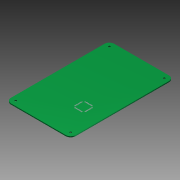
# Autodesk Inventor part: Base station. Board
Saved by Autodesk Inventor 2011 (Build 150239000, 239)
## iProperties
Created: 2011-04-11
Part Number: Base station. Board
Document SubType Name: Modeling
Designer: Rob
Density: 1 g/cm^3
Author: Rob
Autodesk Inventor part; units mm, degrees
ref_plane "YZ Plane" through (0, 0, 0) normal (1, 0, 0) x (0, 1, 0)
ref_plane "XZ Plane" through (0, 0, 0) normal (0, 1, 0) x (-1, 0, 0)
ref_plane "XY Plane" through (0, 0, 0) normal (0, 0, 1) x (1, 0, 0)
sketch "Sketch1" plane through (0, 0, 0) normal (0, 0, 1) x (1, 0, 0)
  line L0 (-50, 80) -> (50, 80)
  line L1 (50, 80) -> (50, -80)
  line L2 (50, -80) -> (-50, -80)
  line L3 (-50, -80) -> (-50, 80)
  line L4 (0, 0) -> (5.0771, 0)
  line L5 (0, 0) -> (0, -4.8823)
  dimension "d0" = 100
  dimension "d1" = 160
  constraints: 12 end point, 3 perpendicular, 2 parallel, 1 horizontal, 2 other
  measures "d0" distance of L1.end L2.end
  measures "d1" distance of L0.end L1.end
extrude "Extrusion1" add sketch "Sketch1" along normal blind 1.6
fillet "Fillet1" radius 7.5 4 edges at (-50, -80, 0.8) (50, -80, 0.8) (-50, 80, 0.8) (50, 80, 0.8)
sketch "Sketch2" plane through (0, 0, 1.6) normal (0, 0, 1) x (1, 0, 0)
  arc A0 (50, 72.5) -> (42.5, 80) centre (42.5, 72.5) ccw projected
  arc A1 (-42.5, 80) -> (-50, 72.5) centre (-42.5, 72.5) ccw projected
  arc A2 (-50, -72.5) -> (-42.5, -80) centre (-42.5, -72.5) ccw projected
  arc A3 (42.5, -80) -> (50, -72.5) centre (42.5, -72.5) ccw projected
  circle A4 centre (-42.5, 72.5) radius 1.5
  circle A5 centre (-42.5, -72.5) radius 1.5
  circle A6 centre (42.5, -72.5) radius 1.5
  circle A7 centre (42.5, 72.5) radius 1.5
  point P0 (0, 0)
  dimension "d5" = 3
  dimension "d6" = 3
  dimension "d7" = 3
  dimension "d8" = 3
  constraints: 4 centre point, 4 coincident
  measures "d5" diameter of A4
  measures "d6" diameter of A5
  measures "d7" diameter of A6
  measures "d8" diameter of A7
extrude "Extrusion2" cut sketch "Sketch2" against normal through all
sketch "Sketch4" plane through (0, 0, 1.6) normal (0, 0, 1) x (1, 0, 0)
  line L0 (42.5, -80) -> (-42.5, -80) projected
  line L1 (50, 72.5) -> (50, -72.5) projected
  line L2 (9.5, -37) -> (27, -37)
  line L3 (27, -37) -> (27, -19.5)
  line L4 (27, -19.5) -> (9.5, -19.5)
  line L5 (9.5, -19.5) -> (9.5, -37)
  line L6 (12.25, -35.25) -> (24.25, -35.25)
  line L7 (25.25, -34.25) -> (25.25, -22.25)
  line L8 (24.25, -21.25) -> (12.25, -21.25)
  line L9 (11.25, -22.25) -> (11.25, -34.25)
  line L10 (18.25, -31.1458) -> (18.25, -23.2964)
  line L11 (18.25, -28.25) -> (14.0823, -28.25)
  arc A0 (11.25, -34.25) -> (12.25, -35.25) centre (12.25, -34.25) ccw
  arc A1 (12.25, -21.25) -> (11.25, -22.25) centre (12.25, -22.25) ccw
  arc A2 (25.25, -22.25) -> (24.25, -21.25) centre (24.25, -22.25) ccw
  arc A3 (24.25, -35.25) -> (25.25, -34.25) centre (24.25, -34.25) ccw
  line L12 (12.25, -21.25) -> (12.75, -21.25)
  line L13 (12.75, -21.25) -> (12.75, -19.5)
  line L14 (12.75, -19.5) -> (12.25, -19.5)
  line L15 (12.25, -19.5) -> (12.25, -21.25)
  line L16 (24.25, -21.25) -> (23.75, -21.25)
  line L17 (23.75, -19.5) -> (24.25, -19.5)
  line L18 (13.0167, -21.25) -> (13.5167, -21.25)
  line L19 (13.5167, -21.25) -> (13.5167, -19.5)
  line L20 (13.5167, -19.5) -> (13.0167, -19.5)
  line L21 (13.0167, -19.5) -> (13.0167, -21.25)
  line L22 (18.1167, -21.25) -> (17.6167, -21.25)
  line L23 (17.6167, -21.25) -> (17.6167, -19.5)
  line L24 (17.6167, -19.5) -> (18.1167, -19.5)
  line L25 (18.1167, -19.5) -> (18.1167, -21.25)
  line L26 (13.7833, -21.25) -> (14.2833, -21.25)
  line L27 (14.2833, -21.25) -> (14.2833, -19.5)
  line L28 (14.2833, -19.5) -> (13.7833, -19.5)
  line L29 (13.7833, -19.5) -> (13.7833, -21.25)
  line L30 (14.55, -21.25) -> (15.05, -21.25)
  line L31 (15.05, -21.25) -> (15.05, -19.5)
  line L32 (15.05, -19.5) -> (14.55, -19.5)
  line L33 (14.55, -19.5) -> (14.55, -21.25)
  line L34 (15.3167, -21.25) -> (15.8167, -21.25)
  line L35 (15.8167, -21.25) -> (15.8167, -19.5)
  line L36 (15.8167, -19.5) -> (15.3167, -19.5)
  line L37 (15.3167, -19.5) -> (15.3167, -21.25)
  line L38 (16.0833, -21.25) -> (16.5833, -21.25)
  line L39 (16.5833, -21.25) -> (16.5833, -19.5)
  line L40 (16.5833, -19.5) -> (16.0833, -19.5)
  line L41 (16.0833, -19.5) -> (16.0833, -21.25)
  line L42 (16.85, -21.25) -> (17.35, -21.25)
  line L43 (17.35, -21.25) -> (17.35, -19.5)
  line L44 (17.35, -19.5) -> (16.85, -19.5)
  line L45 (16.85, -19.5) -> (16.85, -21.25)
  line L46 (24.25, -21.25) -> (23.75, -21.25)
  line L47 (23.75, -21.25) -> (23.75, -19.5)
  line L48 (23.75, -19.5) -> (24.25, -19.5)
  line L49 (24.25, -19.5) -> (24.25, -21.25)
  line L50 (23.4833, -21.25) -> (22.9833, -21.25)
  line L51 (22.9833, -21.25) -> (22.9833, -19.5)
  line L52 (22.9833, -19.5) -> (23.4833, -19.5)
  line L53 (23.4833, -19.5) -> (23.4833, -21.25)
  line L54 (18.3833, -21.25) -> (18.8833, -21.25)
  line L55 (18.8833, -21.25) -> (18.8833, -19.5)
  line L56 (18.8833, -19.5) -> (18.3833, -19.5)
  line L57 (18.3833, -19.5) -> (18.3833, -21.25)
  line L58 (22.7167, -21.25) -> (22.2167, -21.25)
  line L59 (22.2167, -21.25) -> (22.2167, -19.5)
  line L60 (22.2167, -19.5) -> (22.7167, -19.5)
  line L61 (22.7167, -19.5) -> (22.7167, -21.25)
  line L62 (21.95, -21.25) -> (21.45, -21.25)
  line L63 (21.45, -21.25) -> (21.45, -19.5)
  line L64 (21.45, -19.5) -> (21.95, -19.5)
  line L65 (21.95, -19.5) -> (21.95, -21.25)
  line L66 (21.1833, -21.25) -> (20.6833, -21.25)
  line L67 (20.6833, -21.25) -> (20.6833, -19.5)
  line L68 (20.6833, -19.5) -> (21.1833, -19.5)
  line L69 (21.1833, -19.5) -> (21.1833, -21.25)
  line L70 (20.4167, -21.25) -> (19.9167, -21.25)
  line L71 (19.9167, -21.25) -> (19.9167, -19.5)
  line L72 (19.9167, -19.5) -> (20.4167, -19.5)
  line L73 (20.4167, -19.5) -> (20.4167, -21.25)
  line L74 (19.65, -21.25) -> (19.15, -21.25)
  line L75 (19.15, -21.25) -> (19.15, -19.5)
  line L76 (19.15, -19.5) -> (19.65, -19.5)
  line L77 (19.65, -19.5) -> (19.65, -21.25)
  line L78 (24.25, -35.25) -> (12.25, -35.25)
  line L79 (12.25, -35.25) -> (12.75, -35.25)
  line L80 (12.75, -35.25) -> (12.75, -37)
  line L81 (12.75, -37) -> (12.25, -37)
  line L82 (12.25, -37) -> (12.25, -35.25)
  line L83 (24.25, -35.25) -> (23.75, -35.25)
  line L84 (23.75, -37) -> (24.25, -37)
  line L85 (13.0167, -35.25) -> (13.5167, -35.25)
  line L86 (13.5167, -35.25) -> (13.5167, -37)
  line L87 (13.5167, -37) -> (13.0167, -37)
  line L88 (13.0167, -37) -> (13.0167, -35.25)
  line L89 (18.1167, -35.25) -> (17.6167, -35.25)
  line L90 (17.6167, -35.25) -> (17.6167, -37)
  line L91 (17.6167, -37) -> (18.1167, -37)
  line L92 (18.1167, -37) -> (18.1167, -35.25)
  line L93 (13.7833, -35.25) -> (14.2833, -35.25)
  line L94 (14.2833, -35.25) -> (14.2833, -37)
  line L95 (14.2833, -37) -> (13.7833, -37)
  line L96 (13.7833, -37) -> (13.7833, -35.25)
  line L97 (14.55, -35.25) -> (15.05, -35.25)
  line L98 (15.05, -35.25) -> (15.05, -37)
  line L99 (15.05, -37) -> (14.55, -37)
  line L100 (14.55, -37) -> (14.55, -35.25)
  line L101 (15.3167, -35.25) -> (15.8167, -35.25)
  line L102 (15.8167, -35.25) -> (15.8167, -37)
  line L103 (15.8167, -37) -> (15.3167, -37)
  line L104 (15.3167, -37) -> (15.3167, -35.25)
  line L105 (16.0833, -35.25) -> (16.5833, -35.25)
  line L106 (16.5833, -35.25) -> (16.5833, -37)
  line L107 (16.5833, -37) -> (16.0833, -37)
  line L108 (16.0833, -37) -> (16.0833, -35.25)
  line L109 (16.85, -35.25) -> (17.35, -35.25)
  line L110 (17.35, -35.25) -> (17.35, -37)
  line L111 (17.35, -37) -> (16.85, -37)
  line L112 (16.85, -37) -> (16.85, -35.25)
  line L113 (21.95, -37) -> (21.95, -35.25)
  line L114 (21.45, -37) -> (21.95, -37)
  line L115 (21.95, -35.25) -> (21.45, -35.25)
  line L116 (21.1833, -35.25) -> (20.6833, -35.25)
  line L117 (21.1833, -37) -> (21.1833, -35.25)
  line L118 (20.6833, -35.25) -> (20.6833, -37)
  line L119 (20.6833, -37) -> (21.1833, -37)
  line L120 (21.45, -35.25) -> (21.45, -37)
  line L121 (18.3833, -35.25) -> (18.8833, -35.25)
  line L122 (19.65, -35.25) -> (19.15, -35.25)
  line L123 (20.4167, -35.25) -> (19.9167, -35.25)
  line L124 (18.8833, -35.25) -> (18.8833, -37)
  line L125 (18.8833, -37) -> (18.3833, -37)
  line L126 (18.3833, -37) -> (18.3833, -35.25)
  line L127 (19.15, -35.25) -> (19.15, -37)
  line L128 (19.65, -37) -> (19.65, -35.25)
  line L129 (19.15, -37) -> (19.65, -37)
  line L130 (19.9167, -35.25) -> (19.9167, -37)
  line L131 (20.4167, -37) -> (20.4167, -35.25)
  line L132 (19.9167, -37) -> (20.4167, -37)
  line L133 (24.25, -35.25) -> (23.75, -35.25)
  line L134 (23.75, -35.25) -> (23.75, -37)
  line L135 (23.75, -37) -> (24.25, -37)
  line L136 (22.2167, -35.25) -> (22.2167, -37)
  line L137 (22.7167, -35.25) -> (22.2167, -35.25)
  line L138 (22.2167, -37) -> (22.7167, -37)
  line L139 (22.7167, -37) -> (22.7167, -35.25)
  line L140 (22.9833, -35.25) -> (22.9833, -37)
  line L141 (22.9833, -37) -> (23.4833, -37)
  line L142 (23.4833, -37) -> (23.4833, -35.25)
  line L143 (24.25, -37) -> (24.25, -35.25)
  line L144 (23.4833, -35.25) -> (22.9833, -35.25)
  line L145 (11.25, -34.25) -> (9.5, -34.25)
  line L146 (9.5, -34.25) -> (9.5, -33.75)
  line L147 (9.5, -33.75) -> (11.25, -33.75)
  line L148 (11.25, -33.75) -> (11.25, -34.25)
  line L149 (9.5, -33.4833) -> (11.25, -33.4833)
  line L150 (11.25, -33.4833) -> (11.25, -32.9833)
  line L151 (11.25, -32.9833) -> (9.5, -32.9833)
  line L152 (9.5, -32.9833) -> (9.5, -33.4833)
  line L153 (9.5, -32.7167) -> (11.25, -32.7167)
  line L154 (11.25, -32.7167) -> (11.25, -32.2167)
  line L155 (11.25, -32.2167) -> (9.5, -32.2167)
  line L156 (9.5, -32.2167) -> (9.5, -32.7167)
  line L157 (9.5, -31.95) -> (11.25, -31.95)
  line L158 (11.25, -31.95) -> (11.25, -31.45)
  line L159 (11.25, -31.45) -> (9.5, -31.45)
  line L160 (9.5, -31.45) -> (9.5, -31.95)
  line L161 (9.5, -31.1833) -> (11.25, -31.1833)
  line L162 (11.25, -31.1833) -> (11.25, -30.6833)
  line L163 (11.25, -30.6833) -> (9.5, -30.6833)
  line L164 (9.5, -30.6833) -> (9.5, -31.1833)
  line L165 (9.5, -30.4167) -> (11.25, -30.4167)
  line L166 (11.25, -30.4167) -> (11.25, -29.9167)
  line L167 (11.25, -29.9167) -> (9.5, -29.9167)
  line L168 (9.5, -29.9167) -> (9.5, -30.4167)
  line L169 (9.5, -29.65) -> (11.25, -29.65)
  line L170 (11.25, -29.65) -> (11.25, -29.15)
  line L171 (11.25, -29.15) -> (9.5, -29.15)
  line L172 (9.5, -29.15) -> (9.5, -29.65)
  line L173 (9.5, -28.8833) -> (11.25, -28.8833)
  line L174 (11.25, -28.8833) -> (11.25, -28.3833)
  line L175 (11.25, -28.3833) -> (9.5, -28.3833)
  line L176 (9.5, -28.3833) -> (9.5, -28.8833)
  line L177 (11.25, -22.25) -> (9.5, -22.25)
  line L178 (9.5, -22.25) -> (9.5, -22.75)
  line L179 (9.5, -22.75) -> (11.25, -22.75)
  line L180 (11.25, -22.75) -> (11.25, -22.25)
  line L181 (9.5, -23.0167) -> (11.25, -23.0167)
  line L182 (11.25, -23.0167) -> (11.25, -23.5167)
  line L183 (11.25, -23.5167) -> (9.5, -23.5167)
  line L184 (9.5, -23.5167) -> (9.5, -23.0167)
  line L185 (9.5, -23.7833) -> (11.25, -23.7833)
  line L186 (11.25, -23.7833) -> (11.25, -24.2833)
  line L187 (11.25, -24.2833) -> (9.5, -24.2833)
  line L188 (9.5, -24.2833) -> (9.5, -23.7833)
  line L189 (9.5, -24.55) -> (11.25, -24.55)
  line L190 (11.25, -24.55) -> (11.25, -25.05)
  line L191 (11.25, -25.05) -> (9.5, -25.05)
  line L192 (9.5, -25.05) -> (9.5, -24.55)
  line L193 (9.5, -25.3167) -> (11.25, -25.3167)
  line L194 (11.25, -25.3167) -> (11.25, -25.8167)
  line L195 (11.25, -25.8167) -> (9.5, -25.8167)
  line L196 (9.5, -25.8167) -> (9.5, -25.3167)
  line L197 (9.5, -26.0833) -> (11.25, -26.0833)
  line L198 (11.25, -26.0833) -> (11.25, -26.5833)
  line L199 (11.25, -26.5833) -> (9.5, -26.5833)
  line L200 (9.5, -26.5833) -> (9.5, -26.0833)
  line L201 (9.5, -26.85) -> (11.25, -26.85)
  line L202 (11.25, -26.85) -> (11.25, -27.35)
  line L203 (11.25, -27.35) -> (9.5, -27.35)
  line L204 (9.5, -27.35) -> (9.5, -26.85)
  line L205 (9.5, -27.6167) -> (11.25, -27.6167)
  line L206 (11.25, -27.6167) -> (11.25, -28.1167)
  line L207 (11.25, -28.1167) -> (9.5, -28.1167)
  line L208 (9.5, -28.1167) -> (9.5, -27.6167)
  line L209 (25.25, -22.25) -> (25.25, -34.25)
  line L210 (25.25, -34.25) -> (27, -34.25)
  line L211 (27, -34.25) -> (27, -33.75)
  line L212 (27, -33.75) -> (25.25, -33.75)
  line L213 (25.25, -33.75) -> (25.25, -34.25)
  line L214 (27, -33.4833) -> (25.25, -33.4833)
  line L215 (25.25, -33.4833) -> (25.25, -32.9833)
  line L216 (25.25, -32.9833) -> (27, -32.9833)
  line L217 (27, -32.9833) -> (27, -33.4833)
  line L218 (27, -32.7167) -> (25.25, -32.7167)
  line L219 (25.25, -32.7167) -> (25.25, -32.2167)
  line L220 (25.25, -32.2167) -> (27, -32.2167)
  line L221 (27, -32.2167) -> (27, -32.7167)
  line L222 (27, -31.95) -> (25.25, -31.95)
  line L223 (25.25, -31.95) -> (25.25, -31.45)
  line L224 (25.25, -31.45) -> (27, -31.45)
  line L225 (27, -31.45) -> (27, -31.95)
  line L226 (27, -31.1833) -> (25.25, -31.1833)
  line L227 (25.25, -31.1833) -> (25.25, -30.6833)
  line L228 (25.25, -30.6833) -> (27, -30.6833)
  line L229 (27, -30.6833) -> (27, -31.1833)
  line L230 (27, -30.4167) -> (25.25, -30.4167)
  line L231 (25.25, -30.4167) -> (25.25, -29.9167)
  line L232 (25.25, -29.9167) -> (27, -29.9167)
  line L233 (27, -29.9167) -> (27, -30.4167)
  line L234 (27, -29.65) -> (25.25, -29.65)
  line L235 (25.25, -29.65) -> (25.25, -29.15)
  line L236 (25.25, -29.15) -> (27, -29.15)
  line L237 (27, -29.15) -> (27, -29.65)
  line L238 (27, -28.8833) -> (25.25, -28.8833)
  line L239 (25.25, -28.8833) -> (25.25, -28.3833)
  line L240 (25.25, -28.3833) -> (27, -28.3833)
  line L241 (27, -28.3833) -> (27, -28.8833)
  line L242 (25.25, -22.75) -> (25.25, -22.25)
  line L243 (25.25, -23.0167) -> (25.25, -23.5167)
  line L244 (27, -22.25) -> (27, -22.75)
  line L245 (27, -22.75) -> (25.25, -22.75)
  line L246 (27, -23.0167) -> (25.25, -23.0167)
  line L247 (25.25, -23.7833) -> (25.25, -24.2833)
  line L248 (27, -23.5167) -> (27, -23.0167)
  line L249 (25.25, -23.5167) -> (27, -23.5167)
  line L250 (27, -23.7833) -> (25.25, -23.7833)
  line L251 (25.25, -24.2833) -> (27, -24.2833)
  line L252 (27, -24.2833) -> (27, -23.7833)
  line L253 (27, -24.55) -> (25.25, -24.55)
  line L254 (25.25, -22.25) -> (27, -22.25)
  line L255 (25.25, -24.55) -> (25.25, -25.05)
  line L256 (25.25, -25.05) -> (27, -25.05)
  line L257 (27, -25.3167) -> (25.25, -25.3167)
  line L258 (25.25, -25.3167) -> (25.25, -25.8167)
  line L259 (25.25, -25.8167) -> (27, -25.8167)
  line L260 (27, -25.8167) -> (27, -25.3167)
  line L261 (27, -26.0833) -> (25.25, -26.0833)
  line L262 (25.25, -26.0833) -> (25.25, -26.5833)
  line L263 (27, -26.5833) -> (27, -26.0833)
  line L264 (27, -25.05) -> (27, -24.55)
  line L265 (25.25, -26.5833) -> (27, -26.5833)
  line L266 (27, -26.85) -> (25.25, -26.85)
  line L267 (25.25, -26.85) -> (25.25, -27.35)
  line L268 (27, -27.35) -> (27, -26.85)
  line L269 (25.25, -27.35) -> (27, -27.35)
  line L270 (27, -27.6167) -> (25.25, -27.6167)
  line L271 (25.25, -28.1167) -> (27, -28.1167)
  line L272 (27, -28.1167) -> (27, -27.6167)
  line L273 (25.25, -27.6167) -> (25.25, -28.1167)
  line L274 (18.1167, -19.5) -> (18.1167, -21.25)
  point P0 (0, 0)
  point P1 (25.25, -21.25)
  point P2 (25.25, -35.25)
  point P3 (11.25, -21.25)
  dimension "d11" = 17.5
  dimension "d12" = 17.5
  dimension "d13" = 23
  dimension "d14" = 43
  dimension "d15" = 14
  dimension "d16" = 14
  dimension "d17" = 1
  dimension "d18" = 0.5
  dimension "d19" = 0.5
  dimension "d20" = 0.5
  dimension "d21" = 0.5
  dimension "d22" = 0.5
  dimension "d23" = 0.5
  dimension "d24" = 0.5
  dimension "d25" = 0.5
  dimension "d26" = 0.5
  dimension "d27" = 0.2667
  dimension "d28" = 0.2667
  dimension "d29" = 0.2667
  dimension "d30" = 0.2667
  dimension "d31" = 0.2667
  dimension "d32" = 0.2667
  dimension "d33" = 0.2667
  dimension "d34" = 0.5
  dimension "d35" = 0.5
  dimension "d36" = 0.5
  dimension "d37" = 0.5
  dimension "d38" = 0.5
  dimension "d39" = 0.5
  dimension "d40" = 0.5
  dimension "d41" = 0.5
  dimension "d42" = 0.2667
  dimension "d43" = 0.2667
  dimension "d44" = 0.2667
  dimension "d45" = 0.2667
  dimension "d46" = 0.2667
  dimension "d47" = 0.2667
  dimension "d48" = 0.2667
  constraints: 534 end point, 183 symmetric about line, 37 parallel, 21 horizontal, 20 perpendicular, 8 point on circle, 5 point on line, 4 centre point, 4 tangent, 3 equal radius, 3 vertical, 70 other
  measures "d11" distance of point (9.5, -19.5) L3.end
  measures "d12" distance of L3.end L2.end
  measures "d13" distance between parallel lines of L3 L1
  measures "d14" distance between parallel lines of L0 L2
  measures "d15" distance of point (11.25, -21.25) point (25.25, -21.25)
  measures "d16" distance of point (25.25, -21.25) point (25.25, -35.25)
  measures "d17" radius of A0
  measures "d18" distance of L14.end L13.end
  measures "d19" distance of L17.start L17.end
  measures "d20" distance of L20.end L19.end
  measures "d21" distance of L23.end L24.end
  measures "d22" distance of L28.end L27.end
  measures "d23" distance of L32.end L31.end
  measures "d24" distance of L36.end L35.end
  measures "d25" distance of L40.end L39.end
  measures "d26" distance of L43.end L44.end
  measures "d27" distance between parallel lines of L21 L13
  measures "d28" distance between parallel lines of L29 L19
  measures "d29" distance between parallel lines of L27 L33
  measures "d30" distance between parallel lines of L37 L31
  measures "d31" distance between parallel lines of L41 L35
  measures "d32" distance between parallel lines of L45 L39
  measures "d33" distance between parallel lines of L23 L43
  measures "d34" distance of L145.end L146.end
  measures "d35" distance of L150.end L149.end
  measures "d36" distance of L154.end L153.end
  measures "d37" distance of L158.end L157.end
  measures "d38" distance of L162.end L161.end
  measures "d39" distance of L166.end L165.end
  measures "d40" distance of L170.end L169.end
  measures "d41" distance of L175.end L173.start
  measures "d42" distance between parallel lines of L149 L147
  measures "d43" distance between parallel lines of L153 L151
  measures "d44" distance between parallel lines of L157 L155
  measures "d45" distance between parallel lines of L161 L159
  measures "d46" distance between parallel lines of L165 L163
  measures "d47" distance between parallel lines of L169 L167
  measures "d48" distance between parallel lines of L173 L171
extrude "Atmel Connection" add sketch "Sketch4" along normal blind 0.02 contours L82 L6 L80 L2 | L5 L147 L9 L145 | L88 L6 L86 L2 | L5 L151 L9 L149 | L96 L6 L94 L2 | L5 L155 L9 L153 | L100 L6 L98 L2 | L5 L159 L9 L157 | L104 L6 L102 L2 | L5 L163 L9 L161 | L108 L6 L106 L2 | L5 L167 L9 L165 | L112 L6 L110 L2 | L5 L171 L9 L169 | L90 L6 L92 L2 | L5 L175 L9 L173 | L126 L6 L124 L2 | L5 L205 L9 L207 | L127 L6 L128 L2 | L5 L201 L9 L203 | L130 L6 L131 L2 | L5 L197 L9 L199 | L118 L6 L117 L2 | L5 L193 L9 L195 | L120 L6 L113 L2 | L5 L189 L9 L191 | L136 L6 L139 L2 | L5 L185 L9 L187 | L140 L6 L142 L2 | L5 L181 L9 L183 | L134 L6 L143 L2 | L5 L177 L9 L179 | L210 L7 L212 L3 | L4 L13 L8 L15 | L214 L7 L216 L3 | L4 L19 L8 L21 | L218 L7 L220 L3 | L4 L27 L8 L29 | L222 L7 L224 L3 | L4 L31 L8 L33 | L226 L7 L228 L3 | L4 L35 L8 L37 | L230 L7 L232 L3 | L4 L39 L8 L41 | L234 L7 L236 L3 | L4 L43 L8 L45 | L238 L7 L240 L3 | L4 L25 L8 L23 | L271 L7 L270 L3 | L4 L55 L8 L57 | L269 L7 L266 L3 | L4 L77 L8 L75 | L265 L7 L261 L3 | L4 L73 L8 L71 | L259 L7 L257 L3 | L4 L69 L8 L67 | L256 L7 L253 L3 | L4 L65 L8 L63 | L251 L7 L250 L3 | L4 L61 L8 L59 | L249 L7 L246 L3 | L4 L53 L8 L51 | L245 L7 L254 L3 | L4 L49 L8 L47
equation "\"d28\" = d27"
equation "\"d29\" = d27"
equation "\"d30\" = d27"
equation "\"d31\" = d27"
equation "\"d32\" = d27"
equation "\"d33\" = d27"
equation "\"d42\" = d27"
equation "\"d43\" = d27"
equation "\"d44\" = d27"
equation "\"d45\" = d27"
equation "\"d46\" = d27"
equation "\"d47\" = d27"
equation "\"d48\" = d27"
body "Solid1"
